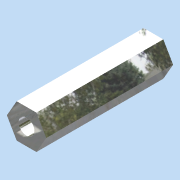
# Autodesk Inventor part: Hex Offset
Saved by Autodesk Inventor 2012 (Build 160160000, 160)
## iProperties
Created: 2012-05-24
Part Number: Hex Offset
Material: Default
Document SubType Name: Modeling
Designer: dgitz
Density: 1 g/cm^3
Author: dgitz
Autodesk Inventor part; units mm, degrees
ref_plane "YZ Plane" through (0, 0, 0) normal (1, 0, 0) x (0, 1, 0)
ref_plane "XZ Plane" through (0, 0, 0) normal (0, 1, 0) x (-1, 0, 0)
ref_plane "XY Plane" through (0, 0, 0) normal (0, 0, 1) x (1, 0, 0)
sketch "Sketch1" plane through (0, 0, 0) normal (0, 0, 1) x (1, 0, 0)
  circle A0 centre (0, 0) radius 1.27
  line L0 (3.1529, 0) -> (1.5765, -2.7305)
  line L1 (1.5765, -2.7305) -> (-1.5765, -2.7305)
  line L2 (-1.5765, -2.7305) -> (-3.1529, 0)
  line L3 (-3.1529, 0) -> (-1.5765, 2.7305)
  line L4 (-1.5765, 2.7305) -> (1.5765, 2.7305)
  line L5 (1.5765, 2.7305) -> (3.1529, 0)
  dimension "d0" = 2.54
  dimension "d1" = 5.461
  constraints: 12 end point, 2 coincident, 1 centre point, 1 horizontal, 13 other
  measures "d0" diameter of A0
  measures "d1" distance between parallel lines of L0 L3
extrude "Extrusion1" add sketch "Sketch1" along normal blind 20.32
body "Solid1"
